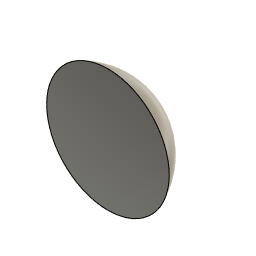
Gimbal (Autodesk Fusion 360 design; units mm, degrees)
Autodesk Fusion 360 part; units mm, degrees
sphere "SpherePrimitive1" add diameter 140 placed x (1, 0, 0) y (0, 1, 0) z (0, 0, 1) at (0, 0, 0) makes body 1
sketch "Sketch3" plane through (0, 0, 0) normal (0, 1, 0) x (1, 0, 0)
  circle A0 centre (0, 0) radius 20
  dimension "d4" = 40
  constraint coincident A0.centre origin
  measures "d4" diameter of A0
extrude "Extrude1" add sketch "Sketch3" against normal blind 150 separate body makes body 2
combine "Combine1" operation cut target body 1 tool bodies 2
sketch "Sketch5" plane through (0, 0, 0) normal (0, 1, 0) x (1, 0, 0)
  line L0 (25, 27) -> (-25, 27)
  line L1 (-25, 27) -> (-25, -27)
  line L2 (-25, -27) -> (25, -27)
  line L3 (25, -27) -> (25, 27)
  line L4 (25, 27) -> (-25, -27) construction
  line L5 (-25, 27) -> (25, -27) construction
  dimension "d7" = 50
  dimension "d8" = 54
  constraint horizontal L0
  constraint perpendicular L0 L1
  constraint parallel L0 L2
  constraint parallel L1 L3
  constraint coincident L4 origin
  constraint coincident L5 origin
  measures "d7" distance of L1.end L2.end
  measures "d8" distance of L0.end L1.end
extrude "Extrude2" add sketch "Sketch5" along normal blind 83 separate body makes body 3
move_body "Move1" bodies 3 to x (1, 0, 0) y (0, 1, 0) z (0, 0, 1) at (0, -70, 0)
move_body "Move2" bodies 3 to x (1, 0, 0) y (0, 1, 0) z (0, 0, 1) at (0, 15, 3.5)
combine "Combine3" operation cut target body 1 tool bodies 3 keep tools
sketch "Sketch7" plane through (0, 0, 0) normal (0, 1, 0) x (-1, 0, 0)
  line L0 (-75, -75) -> (75, -75)
  line L1 (75, -75) -> (75, 75)
  line L2 (75, 75) -> (-75, 75)
  line L3 (-75, 75) -> (-75, -75)
  line L4 (-75, -75) -> (75, 75) construction
  line L5 (75, -75) -> (-75, 75) construction
  dimension "d11" = 150
  dimension "d12" = 150
  constraint horizontal L0
  constraint perpendicular L0 L1
  constraint parallel L0 L2
  constraint parallel L1 L3
  constraint coincident L4 origin
  constraint coincident L5 origin
  measures "d11" distance of L1.end L2.end
  measures "d12" distance of L0.end L1.end
extrude "Extrude3" add sketch "Sketch7" along normal blind 80 separate body makes body 4
move_body "Move3" bodies 4 to x (1, 0, 0) y (0, 1, 0) z (0, 0, 1) at (0, 28, 0)
copy_body "CopyPasteBodies1" bodies 1 makes body 5
combine "Combine4" operation cut target body 1 tool bodies 4 keep tools
sketch "Sketch8" plane through (0, 0, 0) normal (0, 1, 0) x (1, 0, 0)
  line L0 (75, 75) -> (-75, 75)
  line L1 (-75, 75) -> (-75, -75)
  line L2 (-75, -75) -> (75, -75)
  line L3 (75, -75) -> (75, 75)
  line L4 (75, 75) -> (-75, -75) construction
  line L5 (-75, 75) -> (75, -75) construction
  dimension "d15" = 150
  dimension "d16" = 150
  constraint horizontal L0
  constraint perpendicular L0 L1
  constraint parallel L0 L2
  constraint parallel L1 L3
  constraint coincident L4 origin
  constraint coincident L5 origin
  measures "d15" distance of L1.end L2.end
  measures "d16" distance of L0.end L1.end
extrude "Extrude4" add sketch "Sketch8" against normal blind 140 separate body makes body 6
move_body "Move4" bodies 6 to x (1, 0, 0) y (0, 1, 0) z (0, 0, 1) at (0, 28, 0)
combine "Combine5" operation cut target body 5 tool bodies 6 keep tools
sketch "Sketch9" plane through (0, 0, 30.5) normal (0, 0, -1) x (1, 0, 0)
  line L0 (25, 55) -> (-25, 55)
  line L1 (-25, 55) -> (-25, -28)
  line L2 (-25, -28) -> (25, -28)
  line L3 (25, -28) -> (25, 55)
  line L4 (75, 75) -> (-75, 75)
  line L5 (-75, 75) -> (-75, -75)
  line L6 (-75, -75) -> (75, -75)
  line L7 (75, -75) -> (75, 75)
  line L8 (75, 75) -> (-75, -75) construction
  line L9 (-75, 75) -> (75, -75) construction
  dimension "d19" = 150
  dimension "d20" = 150
  constraint horizontal L4
  constraint perpendicular L4 L5
  constraint parallel L4 L6
  constraint parallel L5 L7
  constraint coincident L8 origin
  constraint coincident L9 origin
  measures "d19" distance of L5.end L6.end
  measures "d20" distance of L4.end L5.end
sketch "Sketch10" plane through (0, 0, 0) normal (0, 0, 1) x (1, 0, 0)
  line L0 (75, -75) -> (-75, -75)
  line L1 (-75, -75) -> (-75, 75)
  line L2 (-75, 75) -> (75, 75)
  line L3 (75, 75) -> (75, -75)
  line L4 (75, -75) -> (-75, 75) construction
  line L5 (-75, -75) -> (75, 75) construction
  dimension "d23" = 150
  dimension "d24" = 150
  constraint horizontal L0
  constraint perpendicular L0 L1
  constraint parallel L0 L2
  constraint parallel L1 L3
  constraint coincident L4 origin
  constraint coincident L5 origin
  measures "d23" distance of L1.end L2.end
  measures "d24" distance of L0.end L1.end
extrude "Extrude6" add sketch "Sketch10" against normal blind 75 separate body makes body 7
move_body "Move6" bodies 7 to x (1, 0, 0) y (0, 1, 0) z (0, 0, 1) at (0, 0, -26.5)
copy_body "CopyPasteBodies3" bodies 1 makes body 8
combine "Combine6" operation cut target body 1 tool bodies 7
sketch "Sketch11" plane through (0, 0, 0) normal (0, 0, 1) x (1, 0, 0)
  line L0 (75, -75) -> (-75, -75)
  line L1 (-75, -75) -> (-75, 75)
  line L2 (-75, 75) -> (75, 75)
  line L3 (75, 75) -> (75, -75)
  line L4 (75, -75) -> (-75, 75) construction
  line L5 (-75, -75) -> (75, 75) construction
  dimension "d27" = 150
  dimension "d28" = 150
  constraint horizontal L0
  constraint perpendicular L0 L1
  constraint parallel L0 L2
  constraint parallel L1 L3
  constraint coincident L4 origin
  constraint coincident L5 origin
  measures "d27" distance of L1.end L2.end
  measures "d28" distance of L0.end L1.end
extrude "Extrude7" add sketch "Sketch11" along normal blind 160 separate body makes body 9
move_body "Move7" bodies 9 to x (1, 0, 0) y (0, 1, 0) z (0, 0, 1) at (0, 0, -26.5)
combine "Combine7" operation cut target body 8 tool bodies 9
hidden bodies 1 3 4 6 8
named bodies: "MainBody", "CameraBodyTool", "BodyTool", "RearHatch", "CapTool", "MainBody (1)", "BottomHatch"
